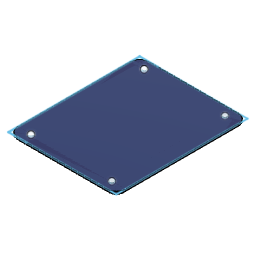
bottom lid (Autodesk Fusion 360 design; units mm, degrees)
Autodesk Fusion 360 part; units mm, degrees
sketch "sketch 407" plane through (0, 0, 108.8238) normal (0, 0, -1) x (0, 1, 0)
  circle A0 centre (81.5775, 46.5972) radius 2
  circle A1 centre (81.5775, 46.5972) radius 2
  circle A2 centre (207.5775, 136.5972) radius 2
  circle A3 centre (81.5775, 136.5972) radius 2
  circle A4 centre (207.5775, 46.5972) radius 2
  circle A5 centre (207.5775, 46.5972) radius 2
  line L0 (71.5775, 151.5972) -> (217.5775, 151.5972)
  line L1 (71.5775, 151.5972) -> (71.5775, 131.5972)
  line L2 (71.5775, 51.5972) -> (71.5775, 131.5972)
  line L3 (71.5775, 31.5972) -> (71.5775, 51.5972)
  line L4 (71.5775, 31.5972) -> (71.5775, 51.5972)
  line L5 (71.5775, 31.5972) -> (217.5775, 31.5972)
  line L6 (71.5775, 31.5972) -> (217.5775, 31.5972)
  line L7 (217.5775, 31.5972) -> (217.5775, 51.5972)
  line L8 (217.5775, 31.5972) -> (217.5775, 51.5972)
  line L9 (217.5775, 51.5972) -> (217.5775, 131.5972)
  line L10 (217.5775, 151.5972) -> (217.5775, 131.5972)
extrude "Extrude1" add sketch "sketch 407" along normal blind 5
fillet "Fillet1" radius 10 4 edges at (31.5972, 217.5775, 106.3238) (31.5972, 71.5775, 106.3238) (151.5972, 71.5775, 106.3238) (151.5972, 217.5775, 106.3238)
chamfer "Chamfer1" distance 3 angle 45 8 edges at (151.5972, 144.5775, 103.8238) (148.6682, 74.5064, 103.8238) (91.5972, 71.5775, 103.8238) (34.5261, 74.5064, 103.8238) (31.5972, 144.5775, 103.8238) (34.5261, 214.6486, 103.8238) (91.5972, 217.5775, 103.8238) (148.6682, 214.6486, 103.8238)
